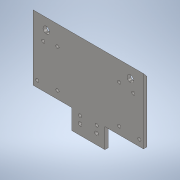
# Autodesk Inventor part: blacha_stal_3mm
Saved by Autodesk Inventor 2022 (Build 260153000, 153)
## iProperties
Created: 2022-12-26
Part Number: blacha_stal_3mm
Material: Steel, Alloy
Document SubType Name: Modeling
Designer: Kamil
Mass: 143.308 g
Surface Area: 137.549 cm^2
Volume: 18.5392 cm^3
Density: 7.73 g/cm^3
Appearance: Semi-Polished
Author: Kamil
Autodesk Inventor part; units mm, degrees
ref_plane "YZ Plane" through (0, 0, 0) normal (1, 0, 0) x (0, 1, 0)
ref_plane "XZ Plane" through (0, 0, 0) normal (0, 1, 0) x (-1, 0, 0)
ref_plane "XY Plane" through (0, 0, 0) normal (0, 0, 1) x (1, 0, 0)
sketch "Sketch1" plane through (0, 0, 0) normal (0, 0, 1) x (1, 0, 0)
  line L0 (15, -2.1558) -> (15, 4.1558) projected
  line L1 (15, 4.1558) -> (-15, 4.1558) projected
  line L2 (-15, 4.1558) -> (-15, -2.1558) projected
  arc A0 (-15, -2.1558) -> (-13, -4.1558) centre (-13, -2.1558) ccw projected
  line L3 (-13, -4.1558) -> (13, -4.1558) projected
  arc A1 (13, -4.1558) -> (15, -2.1558) centre (13, -2.1558) ccw projected
  circle A2 centre (7.5, -0.9558) radius 1.75 projected
  circle A3 centre (-7.5, -0.9558) radius 1.75 projected
  circle A4 centre (7.5, 17.0442) radius 1.75 projected
  line L4 (4.1641, 20.2442) -> (4.1641, 11.9327) projected
  line L5 (4.1641, 11.9327) -> (15, 11.9327) projected
  line L6 (15, 11.9327) -> (15, 18.2442) projected
  arc A5 (15, 18.2442) -> (13, 20.2442) centre (13, 18.2442) ccw projected
  line L7 (13, 20.2442) -> (4.1641, 20.2442) projected
  line L8 (-4.1641, 11.9327) -> (-4.1641, 20.2442) projected
  line L9 (-4.1641, 20.2442) -> (-13, 20.2442) projected
  arc A6 (-13, 20.2442) -> (-15, 18.2442) centre (-13, 18.2442) ccw projected
  line L10 (-15, 18.2442) -> (-15, 11.9327) projected
  line L11 (-15, 11.9327) -> (-4.1641, 11.9327) projected
  circle A7 centre (-7.5, 17.0442) radius 1.75 projected
  line L12 (48, -8.0558) -> (17.2, -8.0558)
  line L13 (-48, -8.0558) -> (-17.2, -8.0558)
  line L14 (48, -8.0558) -> (50, -8.0558)
  line L15 (50, -8.0558) -> (50, 42.8217)
  line L16 (-48, -8.0558) -> (-50, -8.0558)
  line L17 (-50, -8.0558) -> (-50, 42.8217)
  line L18 (50, -8.0558) -> (-50, -8.0558)
  line L19 (-50, -8.0558) -> (-50, 91.9442)
  line L20 (-50, 91.9442) -> (50, 91.9442)
  line L21 (50, 91.9442) -> (50, -8.0558)
  line L22 (48, 24.1442) -> (17.2, 24.1442)
  line L23 (-48, 24.1442) -> (-17.2, 24.1442)
  line L24 (48, 24.1442) -> (17.2, 24.1442)
  line L25 (17.2, 24.1442) -> (17.2, 26.1442)
  line L26 (17.2, 26.1442) -> (48, 26.1442)
  line L27 (48, 26.1442) -> (48, 24.1442)
  line L28 (-48, 24.1442) -> (-17.2, 24.1442)
  line L29 (-17.2, 24.1442) -> (-17.2, 26.1442)
  line L30 (-17.2, 26.1442) -> (-48, 26.1442)
  line L31 (-48, 26.1442) -> (-48, 24.1442)
  line L32 (-15, -4.1558) -> (15, -4.1558)
  line L33 (15, -4.1558) -> (15, 49.5694)
  line L34 (15, 49.5694) -> (-15, 49.5694)
  line L35 (-15, 49.5694) -> (-15, -4.1558)
  line L36 (-50, 91.9442) -> (50, 91.9442)
  line L37 (50, 91.9442) -> (50, 26.1442)
  line L38 (50, 26.1442) -> (-50, 26.1442)
  line L39 (-50, 26.1442) -> (-50, 91.9442)
  point P0 (0, 0)
  point P1 (15, 26.1442)
  point P2 (-15, 26.1442)
  dimension "d2" = 100
  dimension "d3" = 2
  dimension "d4" = 2
  constraints: 56 end point, 11 horizontal, 10 parallel, 7 perpendicular, 3 point on line, 8 other
  measures "d2" distance of L18.end L19.end
  measures "d3" distance of L24.end L25.end
  measures "d4" distance of L29.end L28.end
extrude "Extrusion1" add sketch "Sketch1" along normal blind 2 contours A1 L3 A0 L2 L1 L0 | L33 L32 A1 | L1 L35 L11 L8 L9 A6 L38 L33 A5 L7 L4 L5 | L5 L4 L7 A5 L6 | L32 L35 A0 | L10 A6 L9 L8 L11 | L38 L35 L34 L33 | L33 L34 L35 L38 L30 L17 L19 L20 L21 L15 L26
sketch "Sketch2" plane through (0, 0, 2) normal (0, 0, 1) x (1, 0, 0)
  line L0 (15, -4.1558) -> (15, 26.1442) projected
  line L1 (15, 26.1442) -> (50, 26.1442) projected
  line L2 (50, 26.1442) -> (50, 91.9442) projected
  line L3 (50, 91.9442) -> (-50, 91.9442) projected
  line L4 (-50, 91.9442) -> (-50, 26.1442) projected
  line L5 (-50, 26.1442) -> (-15, 26.1442) projected
  line L6 (-15, 26.1442) -> (-15, -4.1558) projected
  line L7 (-15, -4.1558) -> (15, -4.1558) projected
  circle A0 centre (7.5, -0.9558) radius 1.75 projected
  circle A1 centre (-7.5, -0.9558) radius 1.75 projected
  circle A2 centre (7.5, 17.0442) radius 1.75 projected
  circle A3 centre (-7.5, 17.0442) radius 1.75 projected
  point P0 (0, 0)
extrude "Extrusion2" add sketch "Sketch2" along normal blind 7
extrude "Extrusion3" cut sketch "Sketch2" against normal blind 7
extrude "Extrusion4" cut sketch "Sketch2" along normal blind 4
sketch "Sketch3" plane through (0, 0, 6) normal (0, 0, -1) x (-1, 0, 0)
  line L0 (-15, 26.1442) -> (-50, 26.1442) projected
  line L1 (-15, -4.1558) -> (-15, 26.1442) projected
  line L2 (15, -4.1558) -> (-15, -4.1558) projected
  line L3 (15, 26.1442) -> (15, -4.1558) projected
  line L4 (50, 26.1442) -> (15, 26.1442) projected
  line L5 (50, 91.9442) -> (50, 26.1442) projected
  line L6 (-50, 91.9442) -> (50, 91.9442) projected
  line L7 (-50, 26.1442) -> (-50, 91.9442) projected
  circle A0 centre (-7.5, -0.9558) radius 1.75 projected
  circle A1 centre (7.5, -0.9558) radius 1.75 projected
  circle A2 centre (-7.5, 17.0442) radius 1.75 projected
  circle A3 centre (7.5, 17.0442) radius 1.75 projected
  point P0 (0, 0)
extrude "Extrusion5" add sketch "Sketch3" along normal blind 0.5
sketch "Sketch4" plane through (0, 0, 9) normal (0, 0, 1) x (1, 0, 0)
  line L0 (15, 26.1442) -> (50, 26.1442) projected
  line L1 (50, 26.1442) -> (50, 91.9442) projected
  line L2 (50, 91.9442) -> (-50, 91.9442) projected
  line L3 (-50, 91.9442) -> (-50, 26.1442) projected
  line L4 (-50, 26.1442) -> (-15, 26.1442) projected
  line L5 (-15, 26.1442) -> (-15, -4.1558) projected
  line L6 (-15, -4.1558) -> (15, -4.1558) projected
  line L7 (15, -4.1558) -> (15, 26.1442) projected
  circle A0 centre (7.5, -0.9558) radius 1.75 projected
  circle A1 centre (-7.5, -0.9558) radius 1.75 projected
  circle A2 centre (7.5, 17.0442) radius 1.75 projected
  circle A3 centre (-7.5, 17.0442) radius 1.75 projected
  point P0 (0, 0)
extrude "Extrusion6" cut sketch "Sketch4" against normal blind 0.5
sketch "Sketch5" plane through (0, 0, 5.5) normal (0, 0, -1) x (-1, 0, 0)
  line L0 (-15, -4.1558) -> (15, -4.1558) projected
  line L1 (15, -4.1558) -> (15, 26.1442) projected
  line L2 (15, 26.1442) -> (50, 26.1442) projected
  line L3 (50, 26.1442) -> (50, 91.9442) projected
  line L4 (50, 91.9442) -> (-50, 91.9442) projected
  line L5 (-50, 91.9442) -> (-50, 26.1442) projected
  line L6 (-50, 26.1442) -> (-15, 26.1442) projected
  line L7 (-15, 26.1442) -> (-15, -4.1558) projected
  circle A0 centre (7.5, 17.0442) radius 1.75 projected
  circle A1 centre (-7.5, 17.0442) radius 1.75 projected
  circle A2 centre (7.5, -0.9558) radius 1.75 projected
  circle A3 centre (-7.5, -0.9558) radius 1.75 projected
  circle A4 centre (7.5, -0.9558) radius 1.75 projected
  circle A5 centre (7.5, 17.0442) radius 1.75 projected
  line L8 (7.5, -0.9558) -> (7.5, 17.0442)
  line L9 (7.5, 17.0442) -> (7.5, 35.0442)
  line L10 (7.5, 17.0442) -> (-7.5, 17.0442)
  line L11 (-7.5, 17.0442) -> (-7.5, 35.0442)
  line L12 (-7.5, 35.0442) -> (7.5, 35.0442)
  line L13 (7.5, 35.0442) -> (7.5, 17.0442)
  circle A6 centre (7.5, 35.0442) radius 1.5
  circle A7 centre (-7.5, 35.0442) radius 1.5
  point P0 (0, 0)
  dimension "d20" = 18
  dimension "d21" = 3
  dimension "d22" = 3
  constraints: 12 end point, 2 centre point, 2 coincident, 2 parallel, 2 vertical, 1 horizontal, 1 perpendicular
  measures "d20" distance of L8.end L9.end
  measures "d21" diameter of A7
  measures "d22" diameter of A6
extrude "Extrusion7" cut sketch "Sketch5" against normal through all contours A6 L12 L9 | L9 L12 A6 | A7 L11 L12 | L12 L11 A7
sketch "Sketch6" plane through (15, -4.1558, 5.5) normal (1, 0, 0) x (0, 0, -1)
  line L0 (-3, 30.3) -> (-3, 0) projected
  line L1 (0, 0) -> (-3, 0) projected
  line L2 (0, 30.3) -> (0, 0) projected
  line L3 (0, 30.3) -> (-3, 30.3) projected
  circle A0 centre (11.4185, 12.2) radius 16.1 projected
  line L4 (11.4185, 12.2) -> (-2.2801, 12.2)
  line L5 (-2.2801, 12.2) -> (-8.0401, 12.2)
  circle A1 centre (11.4185, 12.2) radius 14
  point P0 (5.5, 4.1558)
  point P1 (0, 12.2)
  point P2 (-3, 12.2)
  constraints: 4 end point, 1 centre point, 1 coincident, 1 horizontal, 1 point on line
extrude "Extrusion8" cut sketch "Sketch6" against normal through all contours L5 A1 L2 A0 L0 | A0 L2 L1 L0 | L5 L4 L2 A1 picked at (-1.4712, 5.246) picked at (-0.4712, 7.6339)
sketch "Sketch7" plane through (-50, 26.1442, 5.5) normal (-1, 0, 0) x (0, 0, 1)
  line L0 (3, 0) -> (3, 65.8) projected
  line L1 (0, 65.8) -> (3, 65.8) projected
  line L2 (0, 0) -> (0, 65.8) projected
  line L3 (0, 0) -> (3, 0) projected
  circle A0 centre (-10.971, -17.5667) radius 16.1 projected
  line L4 (-10.971, -33.6667) -> (-10.971, 66.3333)
  line L5 (5.129, -17.5667) -> (5.129, 92.1533)
  line L6 (-10.971, 66.3333) -> (5.129, 66.3333)
  line L7 (5.129, 66.3333) -> (-7.5989, 53.6054)
  line L8 (-7.5989, 53.6054) -> (-5.4776, 51.4841)
  line L9 (-5.4776, 51.4841) -> (5.129, 62.0907)
  point P0 (-5.5, -26.1442)
  point P1 (0, 56.9617)
  point P2 (3, 59.9617)
  dimension "d27" = 18
  dimension "d28" = 45
  dimension "d29" = 3
  constraints: 12 end point, 2 perpendicular, 2 point on circle, 2 point on line, 2 vertical, 1 parallel, 1 tangent
  measures "d27" distance of L6.end L7.end
  measures "d28" angle of L5 L7
  measures "d29" distance of L7.end L8.end
extrude "Extrusion9" cut sketch "Sketch7" against normal through all contours L9 L2 L7 L0 | L7 L2 L1 L0
sketch "Sketch9" plane through (-50, 26.1442, 5.5) normal (-1, 0, 0) x (0, 0, 1)
  line L0 (3, 59.9617) -> (0, 56.9617) projected
  line L1 (0, 0) -> (0, 56.9617) projected
  line L2 (0, 0) -> (3, 0) projected
  line L3 (3, 0) -> (3, 59.9617) projected
  circle A0 centre (-10.971, -17.5667) radius 16.1 projected
  line L4 (5.129, -17.5667) -> (5.129, 67.8792)
  line L5 (-10.971, -33.6667) -> (-10.971, 66.3333)
  line L6 (-10.971, 66.3333) -> (9.3716, 66.3333)
  line L7 (5.129, 66.3333) -> (-14.1546, 43.352)
  line L8 (-14.1546, 43.352) -> (-11.8565, 41.4236)
  line L9 (-11.8565, 41.4236) -> (5.129, 61.6661)
  point P0 (-5.5, -26.1442)
  point P1 (0, 55.5537)
  point P2 (3, 59.1289)
  dimension "d37" = 100
  dimension "d38" = 30
  dimension "d39" = 40
  dimension "d40" = 3
  constraints: 12 end point, 3 perpendicular, 3 point on line, 2 point on circle, 2 vertical, 1 tangent
  measures "d37" distance of L5.start L5.end
  measures "d38" distance of L7.start L7.end
  measures "d39" angle of L4 L7
  measures "d40" distance of L7.end L8.end
extrude "Extrusion10" cut sketch "Sketch9" against normal through all contours L3 L9 L1 L0
sketch "Sketch10" plane through (0, 0, 8.5) normal (0, 0, 1) x (1, 0, 0)
  line L0 (2.5, -4.1558) -> (-2.5, -4.1558) projected
  line L1 (-2.5, -4.1558) -> (-2.5, 40.0442) projected
  line L2 (-2.5, 40.0442) -> (-18, 40.0442) projected
  line L3 (-18, 40.0442) -> (-18, 28.8774) projected
  line L4 (-18, 28.8774) -> (-41, 28.8774) projected
  line L5 (-41, 28.8774) -> (-41, 59.7543) projected
  line L6 (-41, 59.7543) -> (-35.2556, 59.7543) projected
  line L7 (-35.2556, 59.7543) -> (-35.2556, 69.9737) projected
  line L8 (-35.2556, 69.9737) -> (-41, 69.9737) projected
  line L9 (-41, 69.9737) -> (-41, 78.0016) projected
  line L10 (-41, 78.0016) -> (-28, 78.0016) projected
  line L11 (-28, 78.0016) -> (-28, 69.9737) projected
  line L12 (-28, 69.9737) -> (28, 69.9737) projected
  line L13 (28, 69.9737) -> (28, 78.0016) projected
  line L14 (28, 78.0016) -> (41, 78.0016) projected
  line L15 (41, 78.0016) -> (41, 69.9737) projected
  line L16 (41, 69.9737) -> (35.2556, 69.9737) projected
  line L17 (35.2556, 69.9737) -> (35.2556, 59.7543) projected
  line L18 (35.2556, 59.7543) -> (41, 59.7543) projected
  line L19 (41, 59.7543) -> (41, 28.8774) projected
  line L20 (41, 28.8774) -> (18, 28.8774) projected
  line L21 (18, 28.8774) -> (18, 40.0442) projected
  line L22 (18, 40.0442) -> (2.5, 40.0442) projected
  line L23 (2.5, 40.0442) -> (2.5, -4.1558) projected
  line L24 (14.3503, 58.5833) -> (3.9031, 60.8951) projected
  line L25 (3.9031, 60.8951) -> (3.5574, 59.3328) projected
  line L26 (3.5574, 59.3328) -> (14.0047, 57.0211) projected
  line L27 (14.0047, 57.0211) -> (14.3503, 58.5833) projected
  line L28 (1.2105, 60.9065) -> (-9.235, 58.5864) projected
  line L29 (-9.235, 58.5864) -> (-8.888, 57.0245) projected
  line L30 (-8.888, 57.0245) -> (1.5574, 59.3445) projected
  line L31 (1.5574, 59.3445) -> (1.2105, 60.9065) projected
  line L32 (-31.4357, 55.8588) -> (-32.5559, 57.0012) projected
  line L33 (-32.5559, 57.0012) -> (-40.1958, 49.5097) projected
  line L34 (-40.1958, 49.5097) -> (-39.0755, 48.3673) projected
  line L35 (-39.0755, 48.3673) -> (-31.4357, 55.8588) projected
  line L36 (38.6369, 43.8085) -> (39.7739, 44.9342) projected
  line L37 (39.7739, 44.9342) -> (32.2458, 52.538) projected
  line L38 (32.2458, 52.538) -> (31.1088, 51.4123) projected
  line L39 (31.1088, 51.4123) -> (38.6369, 43.8085) projected
  line L40 (-34.6166, 43.8763) -> (-36.1788, 44.2217) projected
  line L41 (-36.1788, 44.2217) -> (-38.4885, 33.774) projected
  line L42 (-38.4885, 33.774) -> (-36.9263, 33.4286) projected
  line L43 (-36.9263, 33.4286) -> (-34.6166, 43.8763) projected
  line L44 (39.2388, 29.2757) -> (40.8006, 29.6229) projected
  line L45 (40.8006, 29.6229) -> (38.4785, 40.0679) projected
  line L46 (38.4785, 40.0679) -> (36.9167, 39.7207) projected
  line L47 (36.9167, 39.7207) -> (39.2388, 29.2757) projected
  circle A0 centre (7.5, 35.0442) radius 1.5 projected
  circle A1 centre (-7.5, 35.0442) radius 1.5 projected
  circle A2 centre (7.5, 35.0442) radius 1.5 projected
  line L48 (7.5, 35.0442) -> (28.8902, 35.0442)
  line L49 (0, -4.1558) -> (0, 44.2217)
  line L50 (18, 35.0442) -> (21.5, 35.0442)
  circle A3 centre (21.5, 35.0442) radius 1.5
  circle A4 centre (-21.5, 35.0442) radius 1.5
  point P0 (0, 0)
  dimension "d43" = 3.5
  dimension "d44" = 3
  constraints: 6 end point, 3 point on line, 2 centre point, 1 coincident, 1 horizontal, 1 midpoint, 1 symmetric about line, 1 vertical, 1 other
  measures "d43" distance of L50.start L50.end
  measures "d44" diameter of A3
extrude "Extrusion11" cut sketch "Sketch10" against normal through all contours L48 A3 | L48 A3 | A4
sketch "Sketch11" plane through (0, 0, 8.5) normal (0, 0, 1) x (1, 0, 0)
  line L0 (-39.4778, 77.0915) -> (-36.7778, 77.0915) projected
  line L1 (-36.7778, 77.0915) -> (-36.7778, 73.6915) projected
  line L2 (-36.7778, 73.6915) -> (-39.4778, 73.6915) projected
  line L3 (-39.4778, 73.6915) -> (-39.4778, 77.0915) projected
  line L4 (36.7778, 73.6915) -> (36.7778, 77.0915) projected
  line L5 (39.4778, 73.6915) -> (36.7778, 73.6915) projected
  line L6 (39.4778, 77.0915) -> (39.4778, 73.6915) projected
  line L7 (36.7778, 77.0915) -> (39.4778, 77.0915) projected
  circle A0 centre (-21.5, 35.0442) radius 1.5 projected
  circle A1 centre (21.5, 35.0442) radius 1.5 projected
  circle A2 centre (-7.5, 17.0442) radius 1.75 projected
  circle A3 centre (7.5, 17.0442) radius 1.75 projected
  circle A4 centre (-7.5, 35.0442) radius 1.5 projected
  circle A5 centre (7.5, 35.0442) radius 1.5 projected
  line L8 (50, 85.2732) -> (-50, 85.2732) projected
  line L9 (-50, 26.1442) -> (-50, 85.2732) projected
  line L10 (-15, 26.1442) -> (-50, 26.1442) projected
  line L11 (-15, 8.0442) -> (-15, 26.1442) projected
  line L12 (-15, 8.0442) -> (15, 8.0442) projected
  line L13 (15, 26.1442) -> (15, 8.0442) projected
  line L14 (50, 26.1442) -> (15, 26.1442) projected
  line L15 (50, 85.2732) -> (50, 26.1442) projected
  line L16 (50, 85.2732) -> (-50, 85.2732) projected
  line L17 (0, 85.2732) -> (0, 72.794)
  circle A6 centre (-38.1278, 75.3915) radius 3
  circle A7 centre (38.1278, 75.3915) radius 3
  point P0 (0, 0)
  dimension "d47" = 6
  constraints: 2 centre point, 2 end point, 1 midpoint, 1 symmetric about line, 1 vertical, 1 other
  measures "d47" diameter of A6
extrude "Extrusion12" cut sketch "Sketch11" against normal blind 10 contours L0 L1 L2 L3 | L4 L7 L6 L5 | A6 | A7
sketch "Sketch12" plane through (0, 0, 8.5) normal (0, 0, 1) x (1, 0, 0)
  circle A0 centre (38.1278, 75.3915) radius 3 projected
  circle A1 centre (-38.1278, 75.3915) radius 3 projected
  circle A2 centre (-21.5, 35.0442) radius 1.5 projected
  circle A3 centre (21.5, 35.0442) radius 1.5 projected
  circle A4 centre (-7.5, 17.0442) radius 1.75 projected
  circle A5 centre (7.5, 17.0442) radius 1.75 projected
  circle A6 centre (-7.5, 35.0442) radius 1.5 projected
  circle A7 centre (7.5, 35.0442) radius 1.5 projected
  line L0 (50, 85.2732) -> (-50, 85.2732) projected
  line L1 (-50, 26.1442) -> (-50, 85.2732) projected
  line L2 (-15, 26.1442) -> (-50, 26.1442) projected
  line L3 (-15, 8.0442) -> (-15, 26.1442) projected
  line L4 (-15, 8.0442) -> (15, 8.0442) projected
  line L5 (15, 26.1442) -> (15, 8.0442) projected
  line L6 (50, 26.1442) -> (15, 26.1442) projected
  line L7 (50, 85.2732) -> (50, 26.1442) projected
  circle A8 centre (-46.295, 31.843) radius 1.5
  circle A9 centre (-40.8, 65.3628) radius 1.5
  circle A10 centre (40.8, 65.3628) radius 1.5
  circle A11 centre (46.295, 31.843) radius 1.5
  circle A12 centre (-28, 67.3942) radius 1.5
  circle A13 centre (-28, 33.0442) radius 1.5
  circle A14 centre (28, 33.0442) radius 1.5
  circle A15 centre (28, 67.3942) radius 1.5
  point P0 (0, 0)
  constraints: 8 centre point, 16 other
extrude "Extrusion13" cut sketch "Sketch12" against normal blind 10 contours A8 | A9 | A10 | A11 | A12 | A13 | A14 | A15
ref_plane "Work Plane1" through (36.05, 26.643, 5.5) normal (0, 0, 1) x (1, 0, 0)
extrude "Extrusion14" add sketch "Sketch12" against normal up to surface (3 mm away) contours A2 | A3 | A6 | A7
sketch "Sketch13" plane through (0, 0, 8.5) normal (0, 0, 1) x (1, 0, 0)
  circle A0 centre (7.5, 23.5442) radius 1.5
  circle A1 centre (-7.5, 23.5442) radius 1.5
  point P0 (0, 0)
  constraints: 2 centre point, 4 other
extrude "Extrusion15" cut sketch "Sketch13" against normal blind 10
sketch "Sketch14" plane through (0, 0, 8.5) normal (0, 0, 1) x (1, 0, 0)
  circle A0 centre (-7.5, 23.5442) radius 1.5 projected
  circle A1 centre (7.5, 23.5442) radius 1.5 projected
  circle A2 centre (28, 67.3942) radius 1.5 projected
  circle A3 centre (-28, 33.0442) radius 1.5 projected
  circle A4 centre (28, 33.0442) radius 1.5 projected
  circle A5 centre (-28, 67.3942) radius 1.5 projected
  circle A6 centre (40.8, 65.3628) radius 1.5 projected
  circle A7 centre (-46.295, 31.843) radius 1.5 projected
  circle A8 centre (46.295, 31.843) radius 1.5 projected
  circle A9 centre (-40.8, 65.3628) radius 1.5 projected
  circle A10 centre (38.1278, 75.3915) radius 3 projected
  circle A11 centre (-38.1278, 75.3915) radius 3 projected
  circle A12 centre (-7.5, 17.0442) radius 1.75 projected
  circle A13 centre (7.5, 17.0442) radius 1.75 projected
  line L0 (50, 85.2732) -> (-50, 85.2732) projected
  line L1 (-50, 26.1442) -> (-50, 85.2732) projected
  line L2 (-15, 26.1442) -> (-50, 26.1442) projected
  line L3 (-15, 8.0442) -> (-15, 26.1442) projected
  line L4 (-15, 8.0442) -> (15, 8.0442) projected
  line L5 (15, 26.1442) -> (15, 8.0442) projected
  line L6 (50, 26.1442) -> (15, 26.1442) projected
  line L7 (50, 85.2732) -> (50, 26.1442) projected
  point P0 (0, 0)
extrude "Extrusion16" add sketch "Sketch14" against normal blind 3 contours A10 | A11
sketch "Sketch15" plane through (0, 0, 8.5) normal (0, 0, 1) x (1, 0, 0)
  line L0 (-38.65, 77.1516) -> (-38.65, 73.7516)
  line L1 (-38.65, 73.7516) -> (-35.95, 73.7516)
  line L2 (38.65, 73.7516) -> (38.65, 76.8016)
  line L3 (35.95, 73.7516) -> (38.65, 73.7516)
  line L4 (-38.65, 73.7516) -> (-35.95, 73.7516)
  line L5 (-35.95, 73.7516) -> (-35.95, 77.1516)
  line L6 (-35.95, 77.1516) -> (-38.65, 77.1516)
  line L7 (-38.65, 77.1516) -> (-38.65, 73.7516)
  line L8 (38.65, 73.7516) -> (35.95, 73.7516)
  line L9 (35.95, 73.7516) -> (35.95, 77.1516)
  line L10 (35.95, 77.1516) -> (38.65, 77.1516)
  line L11 (38.65, 77.1516) -> (38.65, 73.7516)
  circle A0 centre (-7.5, 23.5442) radius 1.5 projected
  circle A1 centre (7.5, 23.5442) radius 1.5 projected
  circle A2 centre (28, 67.3942) radius 1.5 projected
  circle A3 centre (-28, 33.0442) radius 1.5 projected
  circle A4 centre (28, 33.0442) radius 1.5 projected
  circle A5 centre (-28, 67.3942) radius 1.5 projected
  circle A6 centre (40.8, 65.3628) radius 1.5 projected
  circle A7 centre (-46.295, 31.843) radius 1.5 projected
  circle A8 centre (46.295, 31.843) radius 1.5 projected
  circle A9 centre (-40.8, 65.3628) radius 1.5 projected
  circle A10 centre (-7.5, 17.0442) radius 1.75 projected
  circle A11 centre (7.5, 17.0442) radius 1.75 projected
  line L12 (50, 85.2732) -> (-50, 85.2732) projected
  line L13 (-50, 26.1442) -> (-50, 85.2732) projected
  line L14 (-15, 26.1442) -> (-50, 26.1442) projected
  line L15 (-15, 8.0442) -> (-15, 26.1442) projected
  line L16 (-15, 8.0442) -> (15, 8.0442) projected
  line L17 (15, 26.1442) -> (15, 8.0442) projected
  line L18 (50, 26.1442) -> (15, 26.1442) projected
  line L19 (50, 85.2732) -> (50, 26.1442) projected
  line L20 (50, 85.2732) -> (-50, 85.2732) projected
  line L21 (0, 85.2732) -> (0, 80.387)
  circle A12 centre (-37.3, 75.4516) radius 3.5
  circle A13 centre (37.3, 75.4516) radius 3.5
  point P0 (0, 0)
  dimension "d58" = 7
  constraints: 26 end point, 4 horizontal, 4 parallel, 3 vertical, 2 centre point, 2 perpendicular, 1 midpoint, 1 point on line, 1 symmetric about line, 7 other
  measures "d58" diameter of A12
extrude "Extrusion17" cut sketch "Sketch15" against normal blind 3 contours L6 L5 L1 L0 | L3 L9 L10 L11 L2 | A12 | A13
body "Solid1"
